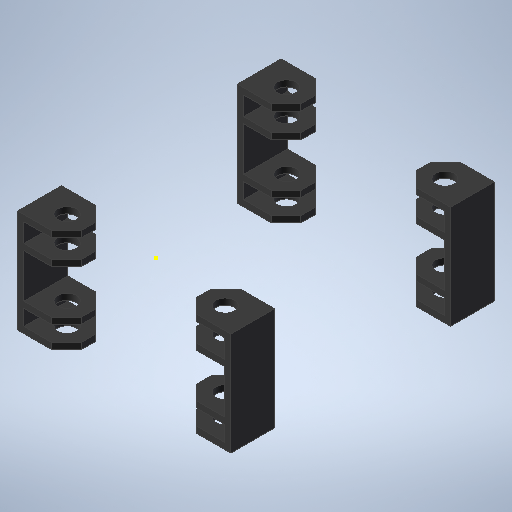
# Autodesk Inventor part: Spacer for PCB boards
Saved by Autodesk Inventor 2025 (Build 290162000, 162)
## iProperties
Created: 2024-07-10
Part Number: Spacer for PCB boards
Material: Generic
Document SubType Name: Modeling
Designer: track
Density: 1 g/cm^3
Appearance: Default
Author: track
## iProperties of the stored document Spacer for PCB boards_3DPrint.ipt
Created: 2024-07-10
Part Number: Spacer for PCB boards_3DPrint
Material: Generic
Document SubType Name: Modeling
Designer: track
Density: 1 g/cm^3
Appearance: Default
Author: track
Autodesk Inventor part; units mm, degrees
ref_plane "YZ Plane" through (0, 0, 0) normal (1, 0, 0) x (0, 1, 0)
ref_plane "XZ Plane" through (0, 0, 0) normal (0, 1, 0) x (-1, 0, 0)
ref_plane "XY Plane" through (0, 0, 0) normal (0, 0, 1) x (1, 0, 0)
sketch "Sketch8" plane through (0, 0, 0) normal (0, 1, 0) x (-1, 0, 0)
  line L0 (-16.05, 21.075) -> (16.05, 21.075)
  line L1 (16.05, 21.075) -> (16.05, -21.075)
  line L2 (16.05, -21.075) -> (-16.05, -21.075)
  line L3 (-16.05, -21.075) -> (-16.05, 21.075)
  line L4 (-16.05, 21.075) -> (16.05, -21.075) construction
  line L5 (16.05, 21.075) -> (-16.05, -21.075) construction
  circle A0 centre (12.65, -17.575) radius 1.5
  line L6 (12.65, -19.075) -> (12.65, -21.075) construction
  line L7 (14.15, -17.575) -> (16.05, -17.575) construction
  line L8 (12.65, -17.575) -> (12.65, -19.075) construction
  line L9 (12.65, -17.575) -> (14.15, -17.575) construction
  line L10 (0, -21.075) -> (0, 21.075) construction
  line L11 (16.05, 0) -> (-16.05, 0) construction
  line L12 (9.25, -14.075) -> (16.05, -14.075)
  line L13 (16.05, -14.075) -> (16.05, -21.075)
  line L14 (16.05, -21.075) -> (9.25, -21.075)
  line L15 (9.25, -21.075) -> (9.25, -14.075)
  line L16 (9.25, -14.075) -> (16.05, -21.075) construction
  line L17 (16.05, -14.075) -> (9.25, -21.075) construction
  circle A1 centre (-12.65, -17.575) radius 1.5
  line L18 (-9.25, -14.075) -> (-16.05, -14.075)
  line L19 (-9.25, -21.075) -> (-9.25, -14.075)
  circle A2 centre (12.65, 17.575) radius 1.5
  line L20 (9.25, 14.075) -> (16.05, 14.075)
  line L21 (9.25, 21.075) -> (9.25, 14.075)
  line L22 (-9.25, 21.075) -> (-9.25, 14.075)
  circle A3 centre (-12.65, 17.575) radius 1.5
  line L23 (-9.25, 14.075) -> (-16.05, 14.075)
  line L24 (16.05, -21.075) -> (22.85, -21.075)
  line L25 (22.85, -21.075) -> (22.85, -14.075)
  line L26 (22.85, -14.075) -> (16.05, -14.075)
  line L27 (16.05, -14.075) -> (16.05, -21.075)
  line L28 (-16.05, -21.075) -> (-22.85, -21.075)
  line L29 (-22.85, -21.075) -> (-22.85, -14.075)
  line L30 (-22.85, -14.075) -> (-16.05, -14.075)
  line L31 (16.05, 21.075) -> (22.85, 21.075)
  line L32 (22.85, 21.075) -> (22.85, 14.075)
  line L33 (22.85, 14.075) -> (16.05, 14.075)
  line L34 (-16.05, 21.075) -> (-22.85, 21.075)
  line L35 (-22.85, 21.075) -> (-22.85, 14.075)
  line L36 (-22.85, 14.075) -> (-16.05, 14.075)
  point P0 (0, 0)
  dimension "d65" = 42.15
  dimension "d66" = 32.1
  dimension "d67" = 3
  dimension "d69" = 2
  dimension "d70" = 1.9
  constraints: 74 end point, 21 symmetric about line, 8 midpoint, 6 parallel, 5 perpendicular, 4 centre point, 3 horizontal, 3 point on circle, 2 collinear, 2 equal length, 2 point on line, 3 other
  measures "d65" distance of L2.end L0.start
  measures "d66" distance of L1.end L2.end
  measures "d67" diameter of A0
  measures "d69" distance of L6.start L6.end
  measures "d70" distance of L7.start L7.end
extrude "Extrusion4" add sketch "Sketch8" along normal blind 1 contours L0 L22 L23 L3 | L3 L36 L35 L34 | L0 L1 L20 L21 | L18 L19 L2 L3 | L3 L28 L29 L30 | L31 L32 L33 L1 | L26 L25 L24 L1 | L1 L2 L15 L12
sketch "Sketch9" plane through (0, 1, 0) normal (0, 1, 0) x (1, 0, 0)
  line L0 (-22.85, 21.075) -> (-22.85, 14.075) projected
  line L1 (-22.85, 21.075) -> (-16.05, 21.075)
  line L2 (-16.05, 21.075) -> (-16.05, 14.075)
  line L3 (-16.05, 14.075) -> (-22.85, 14.075)
  line L4 (-22.85, 14.075) -> (-22.85, 21.075)
  line L5 (-9.25, 21.075) -> (-22.85, 21.075) projected
  line L6 (-16.05, 21.075) -> (-16.05, 14.075) construction
  line L7 (-22.85, 14.075) -> (-9.25, 14.075) projected
  line L8 (0, 20.6342) -> (0, -21.4805) construction
  line L9 (-22.8069, 0) -> (21.3685, 0) construction
  line L10 (22.85, 21.075) -> (22.85, 14.075)
  line L11 (22.85, 21.075) -> (16.05, 21.075)
  line L12 (16.05, 21.075) -> (16.05, 14.075)
  line L13 (16.05, 14.075) -> (22.85, 14.075)
  line L14 (22.85, 14.075) -> (22.85, 21.075)
  line L15 (16.05, 21.075) -> (22.85, 21.075)
  line L16 (22.85, 14.075) -> (16.05, 14.075)
  line L17 (-22.85, -21.075) -> (-22.85, -14.075)
  line L18 (-22.85, -21.075) -> (-16.05, -21.075)
  line L19 (-16.05, -21.075) -> (-16.05, -14.075)
  line L20 (-16.05, -14.075) -> (-22.85, -14.075)
  line L21 (-22.85, -14.075) -> (-22.85, -21.075)
  line L22 (-16.05, -21.075) -> (-22.85, -21.075)
  line L23 (-16.05, -21.075) -> (-16.05, -14.075) construction
  line L24 (-22.85, -14.075) -> (-16.05, -14.075)
  line L25 (0, -20.6342) -> (0, 21.4805) construction
  line L26 (22.85, -21.075) -> (22.85, -14.075)
  line L27 (22.85, -21.075) -> (16.05, -21.075)
  line L28 (16.05, -14.075) -> (22.85, -14.075)
  line L29 (22.85, -14.075) -> (22.85, -21.075)
  line L30 (16.05, -21.075) -> (22.85, -21.075)
  line L31 (22.85, -14.075) -> (16.05, -14.075)
  line L32 (16.05, -21.075) -> (16.05, -14.075)
  point P0 (0, 0)
  point P1 (9.25, 21.075)
  point P2 (9.25, 14.075)
  point P3 (-9.25, -21.075)
  point P4 (-9.25, -14.075)
  point P5 (9.25, -21.075)
  point P6 (9.25, -14.075)
  dimension "d73" = 0
  dimension "d74" = 0
  constraints: 60 end point, 25 symmetric about line, 2 collinear, 2 horizontal, 2 midpoint, 2 parallel, 1 perpendicular, 1 vertical
  measures "d73" distance from line of point (0, 0) L8
  measures "d74" distance from line of point (0, 0) L9
extrude "Extrusion5" add sketch "Sketch9" along normal blind 15.5
sketch "Sketch10" plane through (-16.05, 1, 21.075) normal (1, 0, 0) x (0, 0, -1)
  point P0 (21.075, -1)
sketch "Sketch11" plane through (-16.05, 1, 21.075) normal (1, 0, 0) x (0, 0, -1)
  line L0 (0, 0) -> (0, 15.5) projected
  line L1 (7, 0) -> (7, 15.5) projected
  line L2 (0, 2.5) -> (7, 2.5)
  line L3 (7, 2.5) -> (7, 3.5)
  line L4 (7, 3.5) -> (0, 3.5)
  line L5 (0, 3.5) -> (0, 2.5)
  line L6 (0, -1) -> (7, -1) projected
  line L7 (0, 10.5) -> (7, 10.5)
  line L8 (7, 10.5) -> (7, 11.5)
  line L9 (7, 11.5) -> (0, 11.5)
  line L10 (0, 11.5) -> (0, 10.5)
  line L11 (0, 14.5) -> (7, 14.5)
  line L12 (7, 14.5) -> (7, 15.5)
  line L13 (7, 15.5) -> (0, 15.5)
  line L14 (0, 15.5) -> (0, 14.5)
  line L15 (21.075, -1) -> (21.075, 11.5) construction
  line L16 (42.15, 0) -> (42.15, 15.5)
  line L17 (35.15, 0) -> (35.15, 15.5)
  line L18 (42.15, 2.5) -> (35.15, 2.5)
  line L19 (35.15, 2.5) -> (35.15, 3.5)
  line L20 (35.15, 3.5) -> (42.15, 3.5)
  line L21 (42.15, 3.5) -> (42.15, 2.5)
  line L22 (42.15, -1) -> (35.15, -1)
  line L23 (42.15, 10.5) -> (35.15, 10.5)
  line L24 (35.15, 10.5) -> (35.15, 11.5)
  line L25 (35.15, 11.5) -> (42.15, 11.5)
  line L26 (42.15, 11.5) -> (42.15, 10.5)
  line L27 (42.15, 14.5) -> (35.15, 14.5)
  line L28 (35.15, 14.5) -> (35.15, 15.5)
  line L29 (35.15, 15.5) -> (42.15, 15.5)
  line L30 (42.15, 15.5) -> (42.15, 14.5)
  point P0 (0, 11.5)
  point P1 (7, 10.5)
  point P2 (0, 3.5)
  point P3 (7, 2.5)
  dimension "d77" = 1
  dimension "d78" = 3.5
  dimension "d79" = 1
  dimension "d80" = 1
  dimension "d81" = 7
  dimension "d82" = 3
  constraints: 56 end point, 18 symmetric about line, 12 point on line, 6 parallel, 3 horizontal, 3 perpendicular, 1 vertical
  measures "d77" distance between parallel lines of L4 L2
  measures "d78" distance between parallel lines of L6 L2
  measures "d79" distance between parallel lines of L13 L11
  measures "d80" distance between parallel lines of L9 L7
  measures "d81" distance between parallel lines of L7 L4
  measures "d82" distance between parallel lines of L11 L9
extrude "Extrusion6" add sketch "Sketch11" along normal up to surface (6.8 mm away) contours L0 L4 L1 L2 | L0 L9 L1 L7 | L0 L13 L1 L11 | L18 L17 L20 L16 | L23 L17 L25 L16 | L27 L17 L29 L16
sketch "Sketch12" plane through (16.05, 1, 14.075) normal (-1, 0, 0) x (0, 0, 1)
  line L0 (7, 3.5) -> (0, 3.5) projected
  line L1 (7, 2.5) -> (7, 3.5) projected
  line L2 (0, 2.5) -> (7, 2.5) projected
  line L3 (0, 3.5) -> (0, 2.5) projected
  line L4 (7, 11.5) -> (0, 11.5) projected
  line L5 (7, 10.5) -> (7, 11.5) projected
  line L6 (0, 10.5) -> (7, 10.5) projected
  line L7 (0, 11.5) -> (0, 10.5) projected
  line L8 (7, 15.5) -> (0, 15.5) projected
  line L9 (7, 14.5) -> (7, 15.5) projected
  line L10 (0, 14.5) -> (7, 14.5) projected
  line L11 (0, 15.5) -> (0, 14.5) projected
  line L12 (-28.15, 15.5) -> (-35.15, 15.5) projected
  line L13 (-28.15, 14.5) -> (-28.15, 15.5) projected
  line L14 (-35.15, 14.5) -> (-28.15, 14.5) projected
  line L15 (-35.15, 15.5) -> (-35.15, 14.5) projected
  line L16 (-28.15, 11.5) -> (-35.15, 11.5) projected
  line L17 (-28.15, 10.5) -> (-28.15, 11.5) projected
  line L18 (-35.15, 10.5) -> (-28.15, 10.5) projected
  line L19 (-35.15, 11.5) -> (-35.15, 10.5) projected
  line L20 (-28.15, 2.5) -> (-28.15, 3.5) projected
  line L21 (-35.15, 2.5) -> (-28.15, 2.5) projected
  line L22 (-35.15, 3.5) -> (-35.15, 2.5) projected
  line L23 (-28.15, 3.5) -> (-35.15, 3.5) projected
  point P0 (-14.075, -1)
extrude "Extrusion7" add sketch "Sketch12" along normal up to surface (6.8 mm away)
sketch "Sketch13" plane through (0, 0, 0) normal (0, -1, 0) x (1, 0, 0)
  circle A0 centre (-12.65, -17.575) radius 1.5 projected
  circle A1 centre (-12.65, -17.575) radius 1.5
  line L0 (-22.85, -14.075) -> (-9.25, -14.075) projected
  line L1 (-22.85, -21.075) -> (-9.25, -21.075) projected
  line L2 (-22.85, -14.075) -> (-17.05, -14.075)
  line L3 (-17.05, -14.075) -> (-17.05, -21.075)
  line L4 (-17.05, -21.075) -> (-22.85, -21.075)
  line L5 (-22.85, -21.075) -> (-22.85, -14.075)
  line L6 (-16.05, -21.075) -> (-16.05, -14.075) projected
  line L7 (0, 0) -> (0, -21.075) construction
  line L8 (0, 0) -> (23.0249, 0) construction
  circle A2 centre (12.65, -17.575) radius 1.5
  line L9 (22.85, -14.075) -> (9.25, -14.075)
  line L10 (22.85, -21.075) -> (9.25, -21.075)
  line L11 (22.85, -14.075) -> (17.05, -14.075)
  line L12 (17.05, -14.075) -> (17.05, -21.075)
  line L13 (17.05, -21.075) -> (22.85, -21.075)
  line L14 (22.85, -21.075) -> (22.85, -14.075)
  circle A3 centre (-12.65, 17.575) radius 1.5
  circle A4 centre (-12.65, 17.575) radius 1.5
  line L15 (-22.85, 14.075) -> (-9.25, 14.075)
  line L16 (-22.85, 21.075) -> (-9.25, 21.075)
  line L17 (-22.85, 14.075) -> (-17.05, 14.075)
  line L18 (-17.05, 14.075) -> (-17.05, 21.075)
  line L19 (-17.05, 21.075) -> (-22.85, 21.075)
  line L20 (-22.85, 21.075) -> (-22.85, 14.075)
  line L21 (-16.05, 21.075) -> (-16.05, 14.075)
  line L22 (0, 0) -> (0, 21.075) construction
  circle A5 centre (12.65, 17.575) radius 1.5
  line L23 (22.85, 14.075) -> (9.25, 14.075)
  line L24 (22.85, 21.075) -> (9.25, 21.075)
  line L25 (22.85, 14.075) -> (17.05, 14.075)
  line L26 (17.05, 14.075) -> (17.05, 21.075)
  line L27 (17.05, 21.075) -> (22.85, 21.075)
  line L28 (22.85, 21.075) -> (22.85, 14.075)
  dimension "d87" = 1
  constraints: 52 end point, 28 symmetric about line, 5 centre point, 4 point on line, 2 coincident, 2 horizontal, 2 parallel, 1 perpendicular, 1 vertical, 4 other
  measures "d87" distance between parallel lines of L6 L3
extrude "Extrusion8" cut sketch "Sketch13" against normal through all contours A0 | L0 L3 L1 L5 | A2 | L14 L10 L12 L9 | A3 | L20 L16 L18 L15 | A5 | L23 L26 L24 L28
chamfer "Chamfer2" distance 2.3368 angle 45 32 edges at (-9.25, 16, -14.075) (-9.25, 16, -21.075) (-9.25, 12, -21.075) (-9.25, 12, -14.075) (-9.25, 4, -21.075) (-9.25, 4, -14.075) (-9.25, 0.5, -14.075) (-9.25, 0.5, -21.075) (9.25, 16, -14.075) (9.25, 12, -14.075) (9.25, 4, -14.075) (9.25, 0.5, -14.075) (9.25, 0.5, -21.075) (9.25, 4, -21.075) (9.25, 12, -21.075) (9.25, 16, -21.075) (9.25, 0.5, 14.075) (9.25, 4, 14.075) (9.25, 0.5, 21.075) (9.25, 4, 21.075) (9.25, 12, 14.075) (9.25, 16, 14.075) (9.25, 12, 21.075) (9.25, 16, 21.075) (-9.25, 16, 14.075) (-9.25, 16, 21.075) (-9.25, 12, 14.075) (-9.25, 12, 21.075) (-9.25, 4, 21.075) (-9.25, 4, 14.075) (-9.25, 0.5, 14.075) (-9.25, 0.5, 21.075)
body "Solid2"
